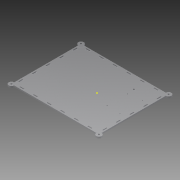
# Autodesk Inventor part: BasePlate2
Saved by Autodesk Inventor 2015 SP1 (Build 190203100, 203)
## iProperties
Created: 2014-08-06
Part Number: BasePlate2
Material: Acrylic, Clear
Document SubType Name: Modeling
Designer: Patrick Camilleri
Density: 1.19 g/cm^3
Appearance: Transparent - Clear
Mass: 654.149 g
Surface Area: 1962.87 cm^2
Volume: 549.705 cm^3
Author: Patrick Camilleri
Autodesk Inventor part; units mm, degrees
ref_plane "YZ Plane" through (0, 0, 0) normal (1, 0, 0) x (0, 1, 0)
ref_plane "XZ Plane" through (0, 0, 0) normal (0, 1, 0) x (-1, 0, 0)
sketch "Sketch1" plane through (0, 0, 0) normal (0, 0, 1) x (1, 0, 0)
  line L0 (-187, -128) -> (135, -128)
  line L1 (135, -128) -> (135, 128)
  line L2 (135, 128) -> (-187, 128)
  line L3 (-187, 128) -> (-187, -128)
  line L4 (-187, 0) -> (135, 0) construction
  line L5 (0, -128) -> (0, 128) construction
  point P0 (0, 0)
  point P1 (0, 0)
  dimension "d160" = 256
  dimension "d161" = 187
  dimension "d162" = 135
  constraints: 12 end point, 3 midpoint, 2 parallel, 2 perpendicular, 2 point on line, 1 coincident, 1 horizontal
  measures "d160" distance of L0.end L1.end
  measures "d161" distance between parallel lines of L3 L5
  measures "d162" distance between parallel lines of L1 L5
extrude "Extrusion1" add sketch "Sketch1" along normal blind 5
sketch "Sketch2" plane through (0, 0, 5) normal (0, 0, 1) x (1, 0, 0)
  line L0 (-182.1, 7.475) -> (-178.9, 7.475)
  line L1 (-178.9, 7.475) -> (-178.9, -7.475)
  line L2 (-178.9, -7.475) -> (-182.1, -7.475)
  line L3 (-182.1, -7.475) -> (-182.1, 7.475)
  line L4 (-182.1, 7.475) -> (-178.9, -7.475) construction
  line L5 (-178.9, 7.475) -> (-182.1, -7.475) construction
  line L6 (-187, -128) -> (135, -128) projected
  line L7 (135, -128) -> (135, 128) projected
  line L8 (135, 128) -> (-187, 128) projected
  line L9 (-187, 128) -> (-187, -128) projected
  line L10 (126.9, -7.475) -> (130.1, -7.475)
  line L11 (130.1, -7.475) -> (130.1, 7.475)
  line L12 (130.1, 7.475) -> (126.9, 7.475)
  line L13 (126.9, 7.475) -> (126.9, -7.475)
  line L14 (126.9, -7.475) -> (130.1, 7.475) construction
  line L15 (130.1, -7.475) -> (126.9, 7.475) construction
  line L16 (-180.5, -121.5) -> (128.5, -121.5) construction
  line L17 (128.5, -121.5) -> (128.5, 121.5) construction
  line L18 (128.5, 121.5) -> (-180.5, 121.5) construction
  line L19 (-180.5, 121.5) -> (-180.5, -121.5) construction
  point P0 (0, 0)
  point P1 (-180.5, 0)
  point P2 (128.5, 0)
  point P3 (128.5, 0)
  point P4 (-180.5, 0)
  dimension "d77" = 3.2
  dimension "d78" = 14.95
  dimension "d163" = 3.2
  dimension "d164" = 14.95
  dimension "d187" = 6.5
  constraints: 32 end point, 8 midpoint, 4 parallel, 2 horizontal, 2 perpendicular, 3 other
  measures "d77" distance of L1.end L2.end
  measures "d78" distance of L0.end L1.end
  measures "d163" distance of L12.end L11.end
  measures "d164" distance of L11.end L10.end
  measures "d187" distance between parallel lines of L9 L19
extrude "Extrusion3" cut sketch "Sketch2" against normal through all contours L0 L1 L2 L3 | L13 L12 L11 L10
sketch "Sketch3" plane through (0, 0, 5) normal (0, 0, 1) x (1, 0, 0)
  line L0 (-162.475, 123.1) -> (-147.525, 123.1)
  line L1 (-147.525, 123.1) -> (-147.525, 119.9)
  line L2 (-147.525, 119.9) -> (-162.475, 119.9)
  line L3 (-162.475, 119.9) -> (-162.475, 123.1)
  line L4 (-162.475, 123.1) -> (-147.525, 119.9) construction
  line L5 (-147.525, 123.1) -> (-162.475, 119.9) construction
  line L6 (-162.475, -119.9) -> (-147.525, -119.9)
  line L7 (-147.525, -119.9) -> (-147.525, -123.1)
  line L8 (-147.525, -123.1) -> (-162.475, -123.1)
  line L9 (-162.475, -123.1) -> (-162.475, -119.9)
  line L10 (-162.475, -119.9) -> (-147.525, -123.1) construction
  line L11 (-147.525, -119.9) -> (-162.475, -123.1) construction
  line L12 (-182.1, -7.475) -> (-182.1, 7.475) projected
  line L13 (-182.1, 7.475) -> (-178.9, 7.475) projected
  line L14 (-178.9, 7.475) -> (-178.9, -7.475) projected
  line L15 (-178.9, -7.475) -> (-182.1, -7.475) projected
  line L16 (-187, -128) -> (135, -128) projected
  line L17 (135, 128) -> (-187, 128) projected
  line L18 (-187, 128) -> (-187, -128) projected
  point P0 (0, 0)
  point P1 (-155, 121.5)
  point P2 (-155, -121.5)
  dimension "d125" = 14.95
  dimension "d126" = 3.2
  dimension "d128" = 14.95
  dimension "d129" = 3.2
  dimension "d198" = 32
  dimension "d199" = 6.5
  dimension "d200" = 32
  dimension "d201" = 6.5
  constraints: 24 end point, 4 midpoint, 4 parallel, 2 horizontal, 2 perpendicular
  measures "d125" distance of L1.end L2.end
  measures "d126" distance of L0.end L1.end
  measures "d128" distance of L7.end L8.end
  measures "d129" distance of L6.end L7.end
  measures "d198" distance from line of L18 point (-155, 121.5)
  measures "d199" distance from line of L17 point (-155, 121.5)
  measures "d200" distance from line of L18 point (-155, -121.5)
  measures "d201" distance from line of L16 point (-155, -121.5)
extrude "Extrusion4" cut sketch "Sketch3" against normal through all contours L0 L1 L2 L3 | L6 L7 L8 L9
pattern_linear "Rectangular Pattern1" count 6 spacing 50 along (1, 0, 0) of "Extrusion4"
pattern_linear "Rectangular Pattern2" count 5 spacing 50 along (0, -1, 0) of "Extrusion3" first direction both ways yes
sketch "Sketch7" plane through (0, 0, 5) normal (0, 0, 1) x (1, 0, 0)
  circle A0 centre (-187, -128) radius 10
  circle A1 centre (135, -128) radius 10
  point P0 (0, 0)
  dimension "d165" = 20
  dimension "d166" = 20
  constraints: 2 centre point, 2 coincident
  measures "d165" diameter of A0
  measures "d166" diameter of A1
extrude "Extrusion6" add sketch "Sketch7" against normal blind 6
mirror "Mirror7" about plane through (0, 0, 0) normal (0, 1, 0) of "Extrusion6"
hole "Hole6" at (-187, -128, 5) direction (0, 0, -1) diameter 6 end through all
hole "Hole7" at (135, -128, 5) direction (0, 0, -1) diameter 6 end through all
mirror "Mirror8" about plane through (0, 0, 0) normal (0, 1, 0) of "Hole6", "Hole7"
sketch "Sketch9" plane through (0, 0, 5) normal (0, 0, 1) x (1, 0, 0)
  line L0 (-178.9, 7.475) -> (-178.9, -7.475) projected
  line L1 (53.25, 82.325) -> (58.2, 82.325)
  line L2 (58.2, 82.325) -> (58.2, 77.475)
  line L3 (58.2, 77.475) -> (53.25, 77.475)
  line L4 (53.25, 77.475) -> (53.25, 82.325)
  line L5 (52.475, 119.9) -> (37.525, 119.9) projected
  point P0 (0, 0)
  point P1 (53.25, 79.9)
  point P2 (53.25, 79.9)
  dimension "d193" = 232.15
  dimension "d194" = 4.95
  dimension "d195" = 4.85
  dimension "d208" = 40
  constraints: 8 end point, 2 parallel, 1 coincident, 1 horizontal, 1 midpoint, 1 perpendicular
  measures "d193" distance from line of point (53.25, 79.9) L0
  measures "d194" distance of L2.end L3.end
  measures "d195" distance of L1.end L2.end
  measures "d208" distance from line of point (53.25, 79.9) L5
extrude "Extrusion8" cut sketch "Sketch9" against normal through all
sketch "Sketch11" plane through (0, 0, 5) normal (0, 0, 1) x (1, 0, 0)
  point P0 (0, 0)
ref_plane "Work Plane1" through (0, 0, 5) normal (0, 1, 0) x (1, 0, 0)
sketch "Sketch14" plane through (0, 0, 5) normal (0, 0, 1) x (1, 0, 0)
  line L0 (52.475, 119.9) -> (37.525, 119.9) projected
  line L1 (126.9, 92.525) -> (126.9, 107.475) projected
  point P0 (0, 0)
  point P1 (106.9, 59.9)
  point P2 (58.64, 53.55)
  point P3 (106.9, -22.65)
  point P4 (58.64, -21.38)
  dimension "d209" = 20
  dimension "d210" = 60
  dimension "d211" = 48.26
  dimension "d212" = 82.55
  dimension "d213" = 74.93
  dimension "d214" = 6.35
  constraints: 2 vertical alignment
  measures "d209" distance from line of point (106.9, 59.9) L1
  measures "d210" distance from line of point (106.9, 59.9) L0
  measures "d211" horizontal distance of point (58.64, 53.55) point (106.9, 59.9)
  measures "d212" distance of point (106.9, -22.65) point (106.9, 59.9)
  measures "d213" distance of point (58.64, -21.38) point (58.64, 53.55)
  measures "d214" vertical distance of point (106.9, 59.9) point (58.64, 53.55)
hole "Hole8" at (58.64, -21.38, 5) at (106.9, -22.65, 5) at (58.64, 53.55, 5) at (106.9, 59.9, 5) direction (0, 0, -1) diameter 3 end through all
equation "\"d166\" = d165"
equation "\"kerf\" = 0.15"
equation "\"slot_w\" = 3.35"
equation "\"slot_l\" = 15.1"
body "Solid1"
